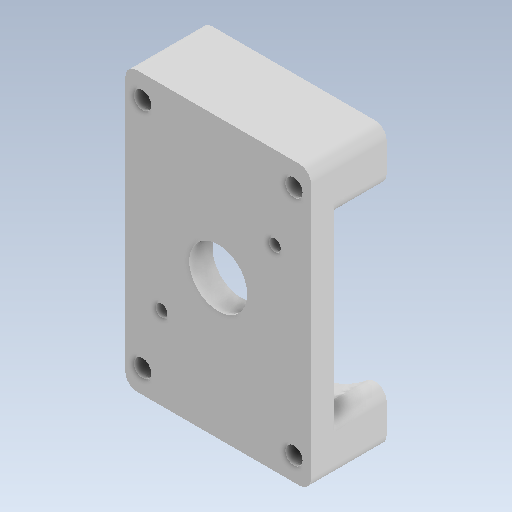
# Autodesk Inventor part: Printed Encoder Mount
Saved by Autodesk Inventor 2020 (Build 240168000, 168)
## iProperties
Created: 2020-03-22
Part Number: Printed Encoder Mount
Material: Generic
Document SubType Name: Modeling
Designer: DasNick
Density: 1 g/cm^3
Appearance: Default
Author: DasNick
Autodesk Inventor part; units mm, degrees
ref_plane "YZ Plane" through (0, 0, 0) normal (1, 0, 0) x (0, 1, 0)
ref_plane "XZ Plane" through (0, 0, 0) normal (0, 1, 0) x (-1, 0, 0)
sketch "Sketch1" plane through (0, 0, 0) normal (0, 0, 1) x (1, 0, 0)
  circle A0 centre (0, 0) radius 31.75 projected
  line L0 (25.4, 38.1) -> (25.4, -38.1) projected
  circle A1 centre (20.7166, 31.75) radius 2.3813 projected
  line L1 (14.986, 531.4221) -> (14.986, -382.9779) projected
  line L2 (-25.4, 38.1) -> (25.4, 38.1) projected
  circle A2 centre (-20.7166, 31.75) radius 2.3813 projected
  line L3 (-25.4, -38.1) -> (-25.4, 38.1) projected
  circle A3 centre (-20.7166, -31.75) radius 2.3813 projected
  line L4 (25.4, -38.1) -> (-25.4, -38.1) projected
  circle A4 centre (20.7166, -31.75) radius 2.3813 projected
  circle A5 centre (0, 0) radius 31.75 projected
  point P0 (0, 0)
  point P1 (25.4, -19.05)
  point P2 (-25.4, -19.05)
  point P3 (-25.4, 19.05)
  point P4 (25.4, 19.05)
ref_plane "Work Plane1" through (-19.4127, -19.4127, 20.695) normal (0, 0, -1) x (0, 1, 0)
extrude "Extrusion1" add sketch "Sketch1" along normal up to surface (20.695 mm away) contours A0 L1 L2 L0 | L0 L4 L1 A0 | A0 L3 L2 L1 | L1 L4 L3 A0
sketch "Sketch2" plane through (0, 0, 20.695) normal (0, 0, 1) x (1, 0, 0)
  arc A0 (-25.4, -19.05) -> (25.4, -19.05) centre (0, 0) ccw projected
  line L0 (25.4, 38.1) -> (25.4, -38.1) projected
  arc A1 (25.4, 19.05) -> (-25.4, 19.05) centre (0, 0) ccw projected
  line L1 (-25.4, -38.1) -> (-25.4, 38.1) projected
  circle A2 centre (-15.5, -15.5) radius 1.6449 projected
  circle A3 centre (15.5, 15.5) radius 1.6449 projected
  circle A4 centre (0, 0) radius 7.9375
  point P0 (0, 0)
  dimension "d2" = 15.875
  constraints: 1 centre point, 1 coincident
  measures "d2" diameter of A4
extrude "Extrusion2" add sketch "Sketch2" against normal blind 6.35
fillet "Fillet1" radius 3.175 8 edges at (-25.4, -19.05, 7.1725) (-25.4, 19.05, 7.1725) (-25.4, 38.1, 10.3475) (25.4, 38.1, 10.3475) (25.4, -38.1, 10.3475) (-25.4, -38.1, 10.3475) (25.4, 19.05, 7.1725) (25.4, -19.05, 7.1725)
body "Solid1"
